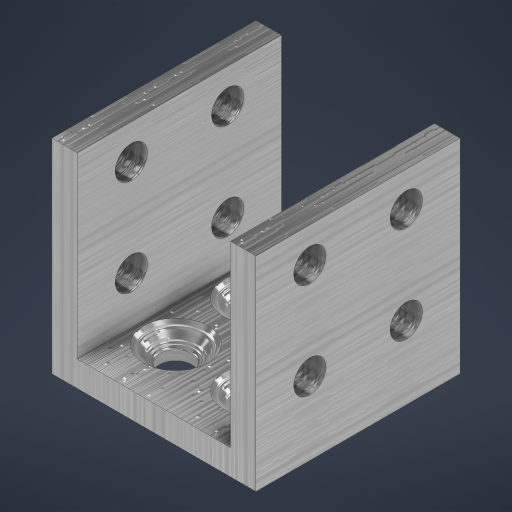
# Autodesk Inventor part: Arashtrix 1in x 1in C-Bracket
Saved by Autodesk Inventor 2024 (Build 280153000, 153)
## iProperties
Created: 2023-11-22
Part Number: Arashtrix 1in x 1in C-Bracket
Material: Generic
Document SubType Name: Modeling
Designer: avsar
Density: 1 g/cm^3
Appearance: Machined 03(1)
Author: avsar
Autodesk Inventor part; units mm, degrees
ref_plane "YZ Plane" through (0, 0, 0) normal (1, 0, 0) x (0, 1, 0)
ref_plane "XZ Plane" through (0, 0, 0) normal (0, 1, 0) x (-1, 0, 0)
ref_plane "XY Plane" through (0, 0, 0) normal (0, 0, 1) x (1, 0, 0)
sketch "Sketch1" plane through (0, 0, 0) normal (0, 0, 1) x (1, 0, 0)
  line L0 (-12.7, 0) -> (12.7, 0)
  line L1 (-12.7, 0) -> (-12.7, 25.4)
  line L2 (12.7, 0) -> (12.7, 25.4)
  line L3 (-9.525, 25.4) -> (-9.525, 3.175)
  line L4 (-9.525, 3.175) -> (9.525, 3.175)
  line L5 (9.525, 3.175) -> (9.525, 25.4)
  line L6 (-12.7, 25.4) -> (-9.525, 25.4)
  line L7 (9.525, 25.4) -> (12.7, 25.4)
  point P0 (0, 0)
  point P1 (0, 0)
  dimension "d0" = 25.4
  dimension "d1" = 25.4
  dimension "d2" = 25.4
  dimension "d3" = 3.175
  constraints: 16 end point, 2 horizontal, 2 vertical, 1 coincident, 1 collinear, 1 midpoint, 2 other
  measures "d0" distance of L0.start L0.end
  measures "d1" distance of L0.start L1.end
  measures "d2" distance of L0.end L2.end
  measures "d3" distance between parallel lines of L1 L3
extrude "Extrusion1" add sketch "Sketch1" along normal mid plane 25.4
sketch "Sketch2" plane through (-9.525, 3.175, 12.7) normal (0, 1, 0) x (1, 0, 0)
  circle A0 centre (4.525, 17.7) radius 2
  circle A1 centre (4.525, 7.7) radius 2
  circle A2 centre (14.525, 7.7) radius 2
  circle A3 centre (14.525, 17.7) radius 2
  point P0 (9.525, 12.7)
  dimension "d6" = 4
  dimension "d7" = 5
  dimension "d8" = 5
  dimension "d11" = 360
  constraints: 4 centre point, 9 other
  measures "d6" diameter of A0
  measures "d7" horizontal distance of A0.centre point (9.525, 12.7)
  measures "d8" horizontal distance of point (9.525, 12.7) A0.centre
hole "Hole1" at (-5, 3.175, 5) at (-5, 3.175, -5) at (5, 3.175, -5) at (5, 3.175, 5) direction (0, -1, 0) diameter 4 depth 3.175 tip angle 118 countersink diameter 8 countersink angle 90
sketch "Sketch3" plane through (12.7, 0, 12.7) normal (1, 0, 0) x (0, 0, -1)
  line L0 (25.4, 3.175) -> (0, 3.175) construction
  line L1 (0, 25.4) -> (0, 3.175) construction
  line L2 (25.4, 25.4) -> (0, 25.4) construction
  line L3 (25.4, 3.175) -> (25.4, 25.4) construction
  line L4 (25.4, 25.4) -> (0, 25.4) construction
  line L5 (0, 0) -> (0, 25.4) construction
  line L6 (0, 12.7) -> (25.4, 17.4625) construction
  circle A0 centre (6.7, 21.0812) radius 2
  circle A1 centre (6.7, 9.0812) radius 2
  circle A2 centre (18.7, 9.0812) radius 2
  circle A3 centre (18.7, 21.0812) radius 2
  line L7 (25.4, 15.0812) -> (0, 15.0812) construction
  point P0 (12.7, 0)
  point P1 (12.7, 15.0812)
  point P2 (25.4, 14.2875)
  point P3 (12.7, 15.0812)
  dimension "d20" = 4
  dimension "d21" = 6
  dimension "d22" = 6
  dimension "d25" = 360
  dimension "d29" = 0.7937
  constraints: 4 centre point, 4 end point, 4 midpoint, 3 point on line, 1 coincident, 1 perpendicular, 9 other
  measures "d20" diameter of A0
  measures "d21" horizontal distance of point (12.7, 15.081) A0.centre
  measures "d22" horizontal distance of A0.centre point (12.7, 15.081)
  measures "d29" distance of L7.start point (25.4, 14.287)
extrude "Extrusion2" cut sketch "Sketch3" against normal through all
body "Solid1"
